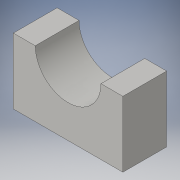
# Autodesk Inventor part: Figure 7_28_10
Saved by Autodesk Inventor 2016 (Build 200138000, 138)
## iProperties
Created: 2016-07-19
Part Number: Figure 7_28_10
Material: Generic
Document SubType Name: Modeling
Designer: cfkguest
Density: 1 g/cm^3
Appearance: Default
Author: cfkguest
Autodesk Inventor part; units mm, degrees
ref_plane "YZ Plane" through (0, 0, 0) normal (1, 0, 0) x (0, 1, 0)
ref_plane "XZ Plane" through (0, 0, 0) normal (0, 1, 0) x (-1, 0, 0)
ref_plane "XY Plane" through (0, 0, 0) normal (0, 0, 1) x (1, 0, 0)
sketch "Sketch1" plane through (0, 0, 0) normal (0, 0, 1) x (1, 0, 0)
  line L0 (-35.7289, 15.5908) -> (27.7711, 15.5908)
  line L1 (27.7711, 15.5908) -> (27.7711, -22.5092)
  line L2 (27.7711, -22.5092) -> (-35.7289, -22.5092)
  line L3 (-35.7289, -22.5092) -> (-35.7289, 15.5908)
  point P0 (0, 0)
  dimension "d0" = 63.5
  dimension "d1" = 38.1
  constraints: 8 end point, 2 parallel, 1 horizontal, 1 perpendicular
  measures "d0" distance of L0.start L0.end
  measures "d1" distance of L0.end L1.end
extrude "Extrusion1" add sketch "Sketch1" along normal blind 25.4
sketch "Sketch2" plane through (0, 0, 25.4) normal (0, 0, 1) x (1, 0, 0)
  line L0 (27.7711, 15.5908) -> (-35.7289, 15.5908) projected
  circle A0 centre (-3.9789, 15.5908) radius 19.05
  point P0 (0, 0)
  dimension "d4" = 38.1
  constraints: 1 centre point, 1 midpoint
  measures "d4" diameter of A0
extrude "Extrusion2" cut sketch "Sketch2" against normal blind 25.4
body "Solid1"
